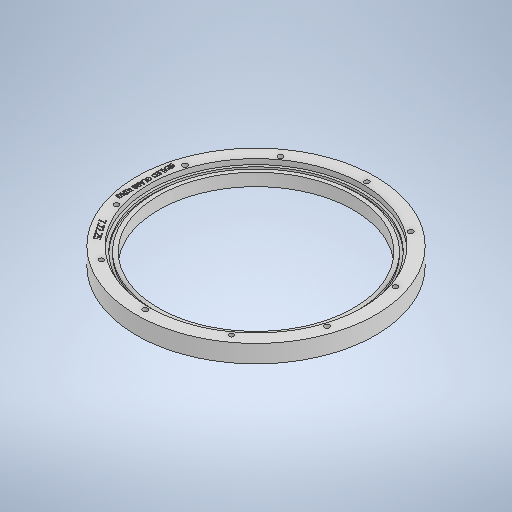
# Autodesk Inventor part: SealedGlassRing
Saved by Autodesk Inventor 2025 (Build 290162000, 162)
## iProperties
Created: 2025-06-19
Part Number: SealedGlassRing
Material: Generic
Document SubType Name: Modeling
Designer: mumin
Density: 1 g/cm^3
Appearance: Default
Author: mumin
Autodesk Inventor part; units mm, degrees
ref_plane "YZ Plane" through (0, 0, 0) normal (1, 0, 0) x (0, 1, 0)
ref_plane "XZ Plane" through (0, 0, 0) normal (0, 1, 0) x (-1, 0, 0)
ref_plane "XY Plane" through (0, 0, 0) normal (0, 0, 1) x (1, 0, 0)
sketch "Sketch1" plane through (0, 0, 0) normal (0, 1, 0) x (-1, 0, 0)
  circle A0 centre (0, 0) radius 110
  circle A1 centre (0, 0) radius 135
  dimension "d0" = 220
  dimension "d1" = 270
  constraints: 2 centre point, 2 coincident
  measures "d0" diameter of A0
  measures "d1" diameter of A1
extrude "Ring" add sketch "Sketch1" along normal blind 20
sketch "Sketch2" plane through (0, 20, 0) normal (0, 1, 0) x (1, 0, 0)
  circle A0 centre (0, 0) radius 120.5
  dimension "d4" = 241
  constraints: 1 centre point, 1 coincident
  measures "d4" diameter of A0
extrude "Glass Seat" cut sketch "Sketch2" against normal blind 5.9
sketch "Sketch3" plane through (0, 20, 0) normal (0, 1, 0) x (1, 0, 0)
  line L0 (0, 189) -> (0, -189) projected
  point P0 (0, 0)
  point P1 (0, 125)
  dimension "d14" = 125
  constraints: 1 point on line
  measures "d14" distance of point (0, 0) point (0, 125)
hole "Holes" at (0, 20, -125) direction (0, -1, 0) diameter 5.5 end through all
pattern_circular "Circular Pattern1" count 10 over 360 about axis through (0, -10, 0) along (0, 1, 0) of "Holes"
sketch "Sketch4" plane through (0, 20, 0) normal (0, 1, 0) x (1, 0, 0)
  line L0 (-123.4008, 33.078) -> (-123.4008, -40.8071) construction
  line L1 (-123.4008, -40.8071) -> (-126.5772, -40.8071) construction
  line L2 (-126.5772, -40.8071) -> (-126.5772, 33.078) construction
  line L3 (-126.5772, 33.078) -> (-123.4008, 33.078) construction
  spline S0 degree 2 poles (-128.5791, 31.1777) (-128.5791, 31.7207) (-128.3522, 32.4824) (-128.1901, 32.8187) knots 0 0 0 1 2 2 2
  line L4 (-128.1901, 32.8187) -> (-127.3554, 32.8187)
  line L5 (-127.3554, 32.8187) -> (-127.3554, 32.7701)
  spline S1 degree 2 poles (-127.3554, 32.7701) (-127.6634, 32.4419) (-128.0037, 31.6113) (-128.0037, 31.2263) knots 0 0 0 1 2 2 2
  spline S2 degree 2 poles (-128.0037, 31.2263) (-128.0037, 30.6753) (-127.5459, 30.1121) (-127.169, 30.1121) knots 0 0 0 1 2 2 2
  spline S3 degree 2 poles (-127.169, 30.1121) (-126.8692, 30.1121) (-126.4964, 30.4079) (-126.4032, 30.7279) knots 0 0 0 1 2 2 2
  spline S4 degree 2 poles (-126.4032, 30.7279) (-126.3384, 30.9589) (-126.2493, 31.3438) (-126.1763, 31.6315) knots 0 0 0 1 2 2 2
  spline S5 degree 2 poles (-126.1763, 31.6315) (-126.1074, 31.8908) (-125.9008, 32.3001) (-125.7347, 32.4581) knots 0 0 0 1 2 2 2
  spline S6 degree 2 poles (-125.7347, 32.4581) (-125.5685, 32.6121) (-125.1228, 32.7822) (-124.8311, 32.7822) knots 0 0 0 1 2 2 2
  spline S7 degree 2 poles (-124.8311, 32.7822) (-124.2233, 32.7822) (-123.4008, 31.8341) (-123.4008, 31.1007) knots 0 0 0 1 2 2 2
  spline S8 degree 2 poles (-123.4008, 31.1007) (-123.4008, 30.6793) (-123.5669, 29.9338) (-123.7249, 29.6137) knots 0 0 0 1 2 2 2
  line L6 (-123.7249, 29.6137) -> (-124.5191, 29.6137)
  line L7 (-124.5191, 29.6137) -> (-124.5191, 29.6623)
  spline S9 degree 2 poles (-124.5191, 29.6623) (-124.3003, 29.9014) (-123.9762, 30.6469) (-123.9762, 31.0561) knots 0 0 0 1 2 2 2
  spline S10 degree 2 poles (-123.9762, 31.0561) (-123.9762, 31.5181) (-124.4097, 32.0894) (-124.7622, 32.0894) knots 0 0 0 1 2 2 2
  spline S11 degree 2 poles (-124.7622, 32.0894) (-125.0783, 32.0894) (-125.4551, 31.7531) (-125.5402, 31.437) knots 0 0 0 1 2 2 2
  spline S12 degree 2 poles (-125.5402, 31.437) (-125.5969, 31.2263) (-125.7428, 30.6145) (-125.8036, 30.4119) knots 0 0 0 1 2 2 2
  spline S13 degree 2 poles (-125.8036, 30.4119) (-125.9616, 29.8973) (-126.5977, 29.4192) (-127.0637, 29.4192) knots 0 0 0 1 2 2 2
  spline S14 degree 2 poles (-127.0637, 29.4192) (-127.3595, 29.4192) (-127.9267, 29.6583) (-128.1253, 29.873) knots 0 0 0 1 2 2 2
  spline S15 degree 2 poles (-128.1253, 29.873) (-128.3441, 30.1121) (-128.5791, 30.7198) (-128.5791, 31.1777) knots 0 0 0 1 2 2 2
  line L8 (-128.4899, 28.7425) -> (-123.4899, 28.7425)
  line L9 (-123.4899, 28.7425) -> (-123.4899, 25.6145)
  line L10 (-123.4899, 25.6145) -> (-124.0815, 25.6145)
  line L11 (-124.0815, 25.6145) -> (-124.0815, 28.078)
  line L12 (-124.0815, 28.078) -> (-125.451, 28.078)
  line L13 (-125.451, 28.078) -> (-125.451, 25.7806)
  line L14 (-125.451, 25.7806) -> (-126.0426, 25.7806)
  line L15 (-126.0426, 25.7806) -> (-126.0426, 28.078)
  line L16 (-126.0426, 28.078) -> (-127.8984, 28.078)
  line L17 (-127.8984, 28.078) -> (-127.8984, 25.6145)
  line L18 (-127.8984, 25.6145) -> (-128.4899, 25.6145)
  line L19 (-128.4899, 25.6145) -> (-128.4899, 28.7425)
  line L20 (-128.4899, 25.4241) -> (-123.4899, 23.7385)
  line L21 (-123.4899, 23.7385) -> (-123.4899, 22.92)
  line L22 (-123.4899, 22.92) -> (-128.4899, 21.2344)
  line L23 (-128.4899, 21.2344) -> (-128.4899, 21.9354)
  line L24 (-128.4899, 21.9354) -> (-127.092, 22.3892)
  line L25 (-127.092, 22.3892) -> (-127.092, 24.2976)
  line L26 (-127.092, 24.2976) -> (-128.4899, 24.7514)
  line L27 (-128.4899, 24.7514) -> (-128.4899, 25.4241)
  line L28 (-126.5248, 22.5715) -> (-124.1707, 23.3455)
  line L29 (-124.1707, 23.3455) -> (-126.5248, 24.1153)
  line L30 (-126.5248, 24.1153) -> (-126.5248, 22.5715)
  line L31 (-128.4899, 17.8633) -> (-128.4899, 20.7604)
  line L32 (-128.4899, 20.7604) -> (-123.4899, 20.7604)
  line L33 (-123.4899, 20.7604) -> (-123.4899, 20.0959)
  line L34 (-123.4899, 20.0959) -> (-127.8984, 20.0959)
  line L35 (-127.8984, 20.0959) -> (-127.8984, 17.8633)
  line L36 (-127.8984, 17.8633) -> (-128.4899, 17.8633)
  line L37 (-128.4899, 17.3406) -> (-123.4899, 17.3406)
  line L38 (-123.4899, 17.3406) -> (-123.4899, 14.2126)
  line L39 (-123.4899, 14.2126) -> (-124.0815, 14.2126)
  line L40 (-124.0815, 14.2126) -> (-124.0815, 16.6761)
  line L41 (-124.0815, 16.6761) -> (-125.451, 16.6761)
  line L42 (-125.451, 16.6761) -> (-125.451, 14.3787)
  line L43 (-125.451, 14.3787) -> (-126.0426, 14.3787)
  line L44 (-126.0426, 14.3787) -> (-126.0426, 16.6761)
  line L45 (-126.0426, 16.6761) -> (-127.8984, 16.6761)
  line L46 (-127.8984, 16.6761) -> (-127.8984, 14.2126)
  line L47 (-127.8984, 14.2126) -> (-128.4899, 14.2126)
  line L48 (-128.4899, 14.2126) -> (-128.4899, 17.3406)
  spline S16 degree 2 poles (-125.994, 9.5408) (-126.6788, 9.5408) (-127.7809, 10.0959) (-128.0888, 10.5618) knots 0 0 0 1 2 2 2
  spline S17 degree 2 poles (-128.0888, 10.5618) (-128.3279, 10.9427) (-128.4899, 11.7247) (-128.4899, 12.3325) knots 0 0 0 1 2 2 2
  line L49 (-128.4899, 12.3325) -> (-128.4899, 13.4832)
  line L50 (-128.4899, 13.4832) -> (-123.4899, 13.4832)
  line L51 (-123.4899, 13.4832) -> (-123.4899, 12.3446)
  spline S18 degree 2 poles (-123.4899, 12.3446) (-123.4899, 11.6396) (-123.7006, 10.8373) (-123.887, 10.5537) knots 0 0 0 1 2 2 2
  spline S19 degree 2 poles (-123.887, 10.5537) (-124.2071, 10.0715) (-125.2647, 9.5408) (-125.994, 9.5408) knots 0 0 0 1 2 2 2
  spline S20 degree 2 poles (-125.9859, 10.2336) (-125.4105, 10.2336) (-124.5961, 10.6145) (-124.3651, 10.9913) knots 0 0 0 1 2 2 2
  spline S21 degree 2 poles (-124.3651, 10.9913) (-124.2071, 11.2587) (-124.0653, 11.8625) (-124.0653, 12.3122) knots 0 0 0 1 2 2 2
  line L52 (-124.0653, 12.3122) -> (-124.0653, 12.8187)
  line L53 (-124.0653, 12.8187) -> (-127.9146, 12.8187)
  line L54 (-127.9146, 12.8187) -> (-127.9146, 12.3122)
  spline S22 degree 2 poles (-127.9146, 12.3122) (-127.9146, 11.8706) (-127.7728, 11.202) (-127.5823, 10.9305) knots 0 0 0 1 2 2 2
  spline S23 degree 2 poles (-127.5823, 10.9305) (-127.3473, 10.5821) (-126.5694, 10.2336) (-125.9859, 10.2336) knots 0 0 0 1 2 2 2
  spline S24 degree 2 poles (-128.5872, 4.5772) (-128.5872, 5.108) (-128.263, 5.9873) (-127.9348, 6.3033) knots 0 0 0 1 2 2 2
  spline S25 degree 2 poles (-127.9348, 6.3033) (-127.6026, 6.6194) (-126.622, 6.9557) (-125.9859, 6.9557) knots 0 0 0 1 2 2 2
  spline S26 degree 2 poles (-125.9859, 6.9557) (-125.3822, 6.9557) (-124.4259, 6.6153) (-124.0856, 6.2993) knots 0 0 0 1 2 2 2
  spline S27 degree 2 poles (-124.0856, 6.2993) (-123.7574, 5.9954) (-123.4008, 5.104) (-123.4008, 4.5732) knots 0 0 0 1 2 2 2
  spline S28 degree 2 poles (-123.4008, 4.5732) (-123.4008, 4.3179) (-123.4737, 3.856) (-123.5386, 3.6453) knots 0 0 0 1 2 2 2
  spline S29 degree 2 poles (-123.5386, 3.6453) (-123.5872, 3.4751) (-123.7655, 3.0618) (-123.8303, 2.9362) knots 0 0 0 1 2 2 2
  line L55 (-123.8303, 2.9362) -> (-124.6326, 2.9362)
  line L56 (-124.6326, 2.9362) -> (-124.6326, 2.9929)
  spline S30 degree 2 poles (-124.6326, 2.9929) (-124.5232, 3.1185) (-124.3246, 3.3819) (-124.2112, 3.625) knots 0 0 0 1 2 2 2
  spline S31 degree 2 poles (-124.2112, 3.625) (-124.1099, 3.8276) (-123.9762, 4.3503) (-123.9762, 4.6502) knots 0 0 0 1 2 2 2
  spline S32 degree 2 poles (-123.9762, 4.6502) (-123.9762, 5.3714) (-125.0621, 6.2628) (-125.9656, 6.2628) knots 0 0 0 1 2 2 2
  spline S33 degree 2 poles (-125.9656, 6.2628) (-126.4681, 6.2628) (-127.2217, 6.0278) (-127.481, 5.8049) knots 0 0 0 1 2 2 2
  spline S34 degree 2 poles (-127.481, 5.8049) (-127.7403, 5.5902) (-128.0118, 4.9824) (-128.0118, 4.6015) knots 0 0 0 1 2 2 2
  spline S35 degree 2 poles (-128.0118, 4.6015) (-128.0118, 4.322) (-127.9308, 3.7628) (-127.8497, 3.5724) knots 0 0 0 1 2 2 2
  line L57 (-127.8497, 3.5724) -> (-126.5572, 3.5724)
  line L58 (-126.5572, 3.5724) -> (-126.5572, 4.7312)
  line L59 (-126.5572, 4.7312) -> (-125.9737, 4.7312)
  line L60 (-125.9737, 4.7312) -> (-125.9737, 2.916)
  line L61 (-125.9737, 2.916) -> (-128.1577, 2.916)
  spline S36 degree 2 poles (-128.1577, 2.916) (-128.2144, 3.0416) (-128.3886, 3.4711) (-128.4413, 3.6534) knots 0 0 0 1 2 2 2
  spline S37 degree 2 poles (-128.4413, 3.6534) (-128.5142, 3.9006) (-128.5872, 4.2976) (-128.5872, 4.5772) knots 0 0 0 1 2 2 2
  line L62 (-128.4899, -0.8158) -> (-128.4899, 2.0813)
  line L63 (-128.4899, 2.0813) -> (-123.4899, 2.0813)
  line L64 (-123.4899, 2.0813) -> (-123.4899, 1.4168)
  line L65 (-123.4899, 1.4168) -> (-127.8984, 1.4168)
  line L66 (-127.8984, 1.4168) -> (-127.8984, -0.8158)
  line L67 (-127.8984, -0.8158) -> (-128.4899, -0.8158)
  line L68 (-128.4899, -0.7996) -> (-123.4899, -2.4852)
  line L69 (-123.4899, -2.4852) -> (-123.4899, -3.3037)
  line L70 (-123.4899, -3.3037) -> (-128.4899, -4.9892)
  line L71 (-128.4899, -4.9892) -> (-128.4899, -4.2883)
  line L72 (-128.4899, -4.2883) -> (-127.092, -3.8345)
  line L73 (-127.092, -3.8345) -> (-127.092, -1.926)
  line L74 (-127.092, -1.926) -> (-128.4899, -1.4722)
  line L75 (-128.4899, -1.4722) -> (-128.4899, -0.7996)
  line L76 (-126.5248, -3.6521) -> (-124.1707, -2.8782)
  line L77 (-124.1707, -2.8782) -> (-126.5248, -2.1084)
  line L78 (-126.5248, -2.1084) -> (-126.5248, -3.6521)
  spline S38 degree 2 poles (-128.5791, -6.8571) (-128.5791, -6.3142) (-128.3522, -5.5524) (-128.1901, -5.2161) knots 0 0 0 1 2 2 2
  line L79 (-128.1901, -5.2161) -> (-127.3554, -5.2161)
  line L80 (-127.3554, -5.2161) -> (-127.3554, -5.2648)
  spline S39 degree 2 poles (-127.3554, -5.2648) (-127.6634, -5.593) (-128.0037, -6.4236) (-128.0037, -6.8085) knots 0 0 0 1 2 2 2
  spline S40 degree 2 poles (-128.0037, -6.8085) (-128.0037, -7.3596) (-127.5459, -7.9228) (-127.169, -7.9228) knots 0 0 0 1 2 2 2
  spline S41 degree 2 poles (-127.169, -7.9228) (-126.8692, -7.9228) (-126.4964, -7.627) (-126.4032, -7.3069) knots 0 0 0 1 2 2 2
  spline S42 degree 2 poles (-126.4032, -7.3069) (-126.3384, -7.0759) (-126.2493, -6.691) (-126.1763, -6.4033) knots 0 0 0 1 2 2 2
  spline S43 degree 2 poles (-126.1763, -6.4033) (-126.1074, -6.144) (-125.9008, -5.7348) (-125.7347, -5.5768) knots 0 0 0 1 2 2 2
  spline S44 degree 2 poles (-125.7347, -5.5768) (-125.5685, -5.4228) (-125.1228, -5.2526) (-124.8311, -5.2526) knots 0 0 0 1 2 2 2
  spline S45 degree 2 poles (-124.8311, -5.2526) (-124.2233, -5.2526) (-123.4008, -6.2007) (-123.4008, -6.9341) knots 0 0 0 1 2 2 2
  spline S46 degree 2 poles (-123.4008, -6.9341) (-123.4008, -7.3555) (-123.5669, -8.1011) (-123.7249, -8.4212) knots 0 0 0 1 2 2 2
  line L81 (-123.7249, -8.4212) -> (-124.5191, -8.4212)
  line L82 (-124.5191, -8.4212) -> (-124.5191, -8.3725)
  spline S47 degree 2 poles (-124.5191, -8.3725) (-124.3003, -8.1335) (-123.9762, -7.3879) (-123.9762, -6.9787) knots 0 0 0 1 2 2 2
  spline S48 degree 2 poles (-123.9762, -6.9787) (-123.9762, -6.5168) (-124.4097, -5.9455) (-124.7622, -5.9455) knots 0 0 0 1 2 2 2
  spline S49 degree 2 poles (-124.7622, -5.9455) (-125.0783, -5.9455) (-125.4551, -6.2818) (-125.5402, -6.5978) knots 0 0 0 1 2 2 2
  spline S50 degree 2 poles (-125.5402, -6.5978) (-125.5969, -6.8085) (-125.7428, -7.4203) (-125.8036, -7.6229) knots 0 0 0 1 2 2 2
  spline S51 degree 2 poles (-125.8036, -7.6229) (-125.9616, -8.1375) (-126.5977, -8.6156) (-127.0637, -8.6156) knots 0 0 0 1 2 2 2
  spline S52 degree 2 poles (-127.0637, -8.6156) (-127.3595, -8.6156) (-127.9267, -8.3766) (-128.1253, -8.1618) knots 0 0 0 1 2 2 2
  spline S53 degree 2 poles (-128.1253, -8.1618) (-128.3441, -7.9228) (-128.5791, -7.315) (-128.5791, -6.8571) knots 0 0 0 1 2 2 2
  spline S54 degree 2 poles (-128.5791, -10.6862) (-128.5791, -10.1432) (-128.3522, -9.3815) (-128.1901, -9.0451) knots 0 0 0 1 2 2 2
  line L83 (-128.1901, -9.0451) -> (-127.3554, -9.0451)
  line L84 (-127.3554, -9.0451) -> (-127.3554, -9.0938)
  spline S55 degree 2 poles (-127.3554, -9.0938) (-127.6634, -9.422) (-128.0037, -10.2526) (-128.0037, -10.6375) knots 0 0 0 1 2 2 2
  spline S56 degree 2 poles (-128.0037, -10.6375) (-128.0037, -11.1886) (-127.5459, -11.7518) (-127.169, -11.7518) knots 0 0 0 1 2 2 2
  spline S57 degree 2 poles (-127.169, -11.7518) (-126.8692, -11.7518) (-126.4964, -11.456) (-126.4032, -11.1359) knots 0 0 0 1 2 2 2
  spline S58 degree 2 poles (-126.4032, -11.1359) (-126.3384, -10.905) (-126.2493, -10.52) (-126.1763, -10.2323) knots 0 0 0 1 2 2 2
  spline S59 degree 2 poles (-126.1763, -10.2323) (-126.1074, -9.973) (-125.9008, -9.5638) (-125.7347, -9.4058) knots 0 0 0 1 2 2 2
  spline S60 degree 2 poles (-125.7347, -9.4058) (-125.5685, -9.2518) (-125.1228, -9.0816) (-124.8311, -9.0816) knots 0 0 0 1 2 2 2
  spline S61 degree 2 poles (-124.8311, -9.0816) (-124.2233, -9.0816) (-123.4008, -10.0298) (-123.4008, -10.7631) knots 0 0 0 1 2 2 2
  spline S62 degree 2 poles (-123.4008, -10.7631) (-123.4008, -11.1845) (-123.5669, -11.9301) (-123.7249, -12.2502) knots 0 0 0 1 2 2 2
  line L85 (-123.7249, -12.2502) -> (-124.5191, -12.2502)
  line L86 (-124.5191, -12.2502) -> (-124.5191, -12.2015)
  spline S63 degree 2 poles (-124.5191, -12.2015) (-124.3003, -11.9625) (-123.9762, -11.2169) (-123.9762, -10.8077) knots 0 0 0 1 2 2 2
  spline S64 degree 2 poles (-123.9762, -10.8077) (-123.9762, -10.3458) (-124.4097, -9.7745) (-124.7622, -9.7745) knots 0 0 0 1 2 2 2
  spline S65 degree 2 poles (-124.7622, -9.7745) (-125.0783, -9.7745) (-125.4551, -10.1108) (-125.5402, -10.4268) knots 0 0 0 1 2 2 2
  spline S66 degree 2 poles (-125.5402, -10.4268) (-125.5969, -10.6375) (-125.7428, -11.2494) (-125.8036, -11.452) knots 0 0 0 1 2 2 2
  spline S67 degree 2 poles (-125.8036, -11.452) (-125.9616, -11.9665) (-126.5977, -12.4447) (-127.0637, -12.4447) knots 0 0 0 1 2 2 2
  spline S68 degree 2 poles (-127.0637, -12.4447) (-127.3595, -12.4447) (-127.9267, -12.2056) (-128.1253, -11.9909) knots 0 0 0 1 2 2 2
  spline S69 degree 2 poles (-128.1253, -11.9909) (-128.3441, -11.7518) (-128.5791, -11.144) (-128.5791, -10.6862) knots 0 0 0 1 2 2 2
  line L87 (-128.4899, -19.1383) -> (-128.4899, -18.2753)
  line L88 (-128.4899, -18.2753) -> (-126.5005, -16.6951)
  line L89 (-126.5005, -16.6951) -> (-126.5005, -15.9333)
  line L90 (-126.5005, -15.9333) -> (-128.4899, -15.9333)
  line L91 (-128.4899, -15.9333) -> (-128.4899, -15.2688)
  line L92 (-128.4899, -15.2688) -> (-123.4899, -15.2688)
  line L93 (-123.4899, -15.2688) -> (-123.4899, -16.5573)
  spline S70 degree 2 poles (-123.4899, -16.5573) (-123.4899, -16.9868) (-123.5831, -17.5662) (-123.7533, -17.8296) knots 0 0 0 1 2 2 2
  spline S71 degree 2 poles (-123.7533, -17.8296) (-123.9235, -18.093) (-124.4543, -18.3968) (-124.8473, -18.3968) knots 0 0 0 1 2 2 2
  spline S72 degree 2 poles (-124.8473, -18.3968) (-125.3943, -18.3968) (-126.1358, -17.8377) (-126.3141, -17.3596) knots 0 0 0 1 2 2 2
  line L94 (-126.3141, -17.3596) -> (-128.4899, -19.1383)
  spline S73 degree 2 poles (-124.9, -17.704) (-124.6812, -17.704) (-124.3449, -17.55) (-124.2355, -17.3879) knots 0 0 0 1 2 2 2
  spline S74 degree 2 poles (-124.2355, -17.3879) (-124.1423, -17.2461) (-124.0653, -16.8693) (-124.0653, -16.5938) knots 0 0 0 1 2 2 2
  line L95 (-124.0653, -16.5938) -> (-124.0653, -15.9333)
  line L96 (-124.0653, -15.9333) -> (-125.9454, -15.9333)
  line L97 (-125.9454, -15.9333) -> (-125.9454, -16.5168)
  spline S75 degree 2 poles (-125.9454, -16.5168) (-125.9454, -16.8045) (-125.8441, -17.2623) (-125.686, -17.4203) knots 0 0 0 1 2 2 2
  spline S76 degree 2 poles (-125.686, -17.4203) (-125.5483, -17.5662) (-125.1593, -17.704) (-124.9, -17.704) knots 0 0 0 1 2 2 2
  line L98 (-128.4899, -21.2777) -> (-128.4899, -19.3409)
  line L99 (-128.4899, -19.3409) -> (-127.9794, -19.3409)
  line L100 (-127.9794, -19.3409) -> (-127.9794, -19.9771)
  line L101 (-127.9794, -19.9771) -> (-124.0005, -19.9771)
  line L102 (-124.0005, -19.9771) -> (-124.0005, -19.3409)
  line L103 (-124.0005, -19.3409) -> (-123.4899, -19.3409)
  line L104 (-123.4899, -19.3409) -> (-123.4899, -21.2777)
  line L105 (-123.4899, -21.2777) -> (-124.0005, -21.2777)
  line L106 (-124.0005, -21.2777) -> (-124.0005, -20.6416)
  line L107 (-124.0005, -20.6416) -> (-127.9794, -20.6416)
  line L108 (-127.9794, -20.6416) -> (-127.9794, -21.2777)
  line L109 (-127.9794, -21.2777) -> (-128.4899, -21.2777)
  line L110 (-128.4899, -25.678) -> (-128.4899, -24.9325)
  line L111 (-128.4899, -24.9325) -> (-124.1788, -22.7202)
  line L112 (-124.1788, -22.7202) -> (-128.4899, -22.7202)
  line L113 (-128.4899, -22.7202) -> (-128.4899, -22.1003)
  line L114 (-128.4899, -22.1003) -> (-123.4899, -22.1003)
  line L115 (-123.4899, -22.1003) -> (-123.4899, -23.0443)
  line L116 (-123.4899, -23.0443) -> (-127.4486, -25.0581)
  line L117 (-127.4486, -25.0581) -> (-123.4899, -25.0581)
  line L118 (-123.4899, -25.0581) -> (-123.4899, -25.678)
  line L119 (-123.4899, -25.678) -> (-128.4899, -25.678)
  spline S77 degree 2 poles (-128.5872, -28.7858) (-128.5872, -28.255) (-128.263, -27.3758) (-127.9348, -27.0597) knots 0 0 0 1 2 2 2
  spline S78 degree 2 poles (-127.9348, -27.0597) (-127.6026, -26.7437) (-126.622, -26.4074) (-125.9859, -26.4074) knots 0 0 0 1 2 2 2
  spline S79 degree 2 poles (-125.9859, -26.4074) (-125.3822, -26.4074) (-124.4259, -26.7477) (-124.0856, -27.0638) knots 0 0 0 1 2 2 2
  spline S80 degree 2 poles (-124.0856, -27.0638) (-123.7574, -27.3677) (-123.4008, -28.2591) (-123.4008, -28.7899) knots 0 0 0 1 2 2 2
  spline S81 degree 2 poles (-123.4008, -28.7899) (-123.4008, -29.0451) (-123.4737, -29.5071) (-123.5386, -29.7178) knots 0 0 0 1 2 2 2
  spline S82 degree 2 poles (-123.5386, -29.7178) (-123.5872, -29.8879) (-123.7655, -30.3012) (-123.8303, -30.4268) knots 0 0 0 1 2 2 2
  line L120 (-123.8303, -30.4268) -> (-124.6326, -30.4268)
  line L121 (-124.6326, -30.4268) -> (-124.6326, -30.3701)
  spline S83 degree 2 poles (-124.6326, -30.3701) (-124.5232, -30.2445) (-124.3246, -29.9811) (-124.2112, -29.738) knots 0 0 0 1 2 2 2
  spline S84 degree 2 poles (-124.2112, -29.738) (-124.1099, -29.5354) (-123.9762, -29.0127) (-123.9762, -28.7129) knots 0 0 0 1 2 2 2
  spline S85 degree 2 poles (-123.9762, -28.7129) (-123.9762, -27.9917) (-125.0621, -27.1003) (-125.9656, -27.1003) knots 0 0 0 1 2 2 2
  spline S86 degree 2 poles (-125.9656, -27.1003) (-126.4681, -27.1003) (-127.2217, -27.3353) (-127.481, -27.5581) knots 0 0 0 1 2 2 2
  spline S87 degree 2 poles (-127.481, -27.5581) (-127.7403, -27.7729) (-128.0118, -28.3806) (-128.0118, -28.7615) knots 0 0 0 1 2 2 2
  spline S88 degree 2 poles (-128.0118, -28.7615) (-128.0118, -29.0411) (-127.9308, -29.6003) (-127.8497, -29.7907) knots 0 0 0 1 2 2 2
  line L122 (-127.8497, -29.7907) -> (-126.5572, -29.7907)
  line L123 (-126.5572, -29.7907) -> (-126.5572, -28.6319)
  line L124 (-126.5572, -28.6319) -> (-125.9737, -28.6319)
  line L125 (-125.9737, -28.6319) -> (-125.9737, -30.4471)
  line L126 (-125.9737, -30.4471) -> (-128.1577, -30.4471)
  spline S89 degree 2 poles (-128.1577, -30.4471) (-128.2144, -30.3215) (-128.3886, -29.892) (-128.4413, -29.7097) knots 0 0 0 1 2 2 2
  spline S90 degree 2 poles (-128.4413, -29.7097) (-128.5142, -29.4625) (-128.5872, -29.0654) (-128.5872, -28.7858) knots 0 0 0 1 2 2 2
  point P0 (0, 0)
  constraints: 2 other
emboss "Emboss1" sketch "Sketch4" operation cut depth 1 direction (0, -1, 0)
sketch "Sketch5" plane through (0, 14.1, 0) normal (0, 1, 0) x (1, 0, 0)
  circle A0 centre (0, 0) radius 120.5 projected
  circle A1 centre (0, 0) radius 117.5
  circle A2 centre (0, 0) radius 114.5
  dimension "d25" = 3
  dimension "d26" = 3
  constraints: 2 centre point
  measures "d25" radial gap between concentric circles of A0 A1
  measures "d26" radial gap between concentric circles of A1 A2
extrude "Seal Groove" cut sketch "Sketch5" against normal blind 2.5 contours A1
sketch "Sketch6" plane through (0, 20, 0) normal (0, 1, 0) x (1, 0, 0)
  line L0 (-109.3924, -58.9981) -> (-82.8013, -97.4436) construction
  line L1 (-82.8013, -97.4436) -> (-85.9073, -99.5919) construction
  line L2 (-85.9073, -99.5919) -> (-112.4984, -61.1464) construction
  line L3 (-112.4984, -61.1464) -> (-109.3924, -58.9981) construction
  line L4 (-107.8437, -63.0408) -> (-113.5155, -63.8067)
  line L5 (-113.5155, -63.8067) -> (-114.0023, -63.1029)
  line L6 (-114.0023, -63.1029) -> (-108.0876, -62.3463)
  line L7 (-108.0876, -62.3463) -> (-109.8494, -59.799)
  line L8 (-109.8494, -59.799) -> (-109.2696, -59.3979)
  line L9 (-109.2696, -59.3979) -> (-107.1039, -62.5291)
  line L10 (-107.1039, -62.5291) -> (-107.8437, -63.0408)
  line L11 (-110.8879, -67.6057) -> (-111.4356, -66.8139)
  line L12 (-111.4356, -66.8139) -> (-110.4918, -66.1612)
  line L13 (-110.4918, -66.1612) -> (-109.9442, -66.953)
  line L14 (-109.9442, -66.953) -> (-110.8879, -67.6057)
  line L15 (-108.0944, -71.6446) -> (-110.1992, -68.6014)
  line L16 (-110.1992, -68.6014) -> (-109.4994, -68.1174)
  spline S0 degree 2 poles (-109.4994, -68.1174) (-108.9647, -68.2323) (-107.989, -68.4207) (-107.4875, -68.4876) knots 0 0 0 1 2 2 2
  spline S1 degree 2 poles (-107.4875, -68.4876) (-106.4777, -68.6227) (-105.449, -68.5202) (-105.0531, -68.2464) knots 0 0 0 1 2 2 2
  spline S2 degree 2 poles (-105.0531, -68.2464) (-104.8452, -68.1025) (-104.6218, -67.7588) (-104.602, -67.5737) knots 0 0 0 1 2 2 2
  spline S3 degree 2 poles (-104.602, -67.5737) (-104.5823, -67.3886) (-104.6925, -67.0155) (-104.8197, -66.8316) knots 0 0 0 1 2 2 2
  spline S4 degree 2 poles (-104.8197, -66.8316) (-104.9414, -66.6556) (-105.2783, -66.3566) (-105.4597, -66.2396) knots 0 0 0 1 2 2 2
  spline S5 degree 2 poles (-105.4597, -66.2396) (-105.6125, -66.1384) (-105.9522, -65.9891) (-106.0635, -65.9479) knots 0 0 0 1 2 2 2
  line L17 (-106.0635, -65.9479) -> (-106.0884, -65.9119)
  line L18 (-106.0884, -65.9119) -> (-105.3846, -65.4251)
  spline S6 degree 2 poles (-105.3846, -65.4251) (-105.1436, -65.5599) (-104.4415, -66.1561) (-104.2147, -66.4841) knots 0 0 0 1 2 2 2
  spline S7 degree 2 poles (-104.2147, -66.4841) (-103.7362, -67.1759) (-103.9286, -68.4618) (-104.5525, -68.8933) knots 0 0 0 1 2 2 2
  spline S8 degree 2 poles (-104.5525, -68.8933) (-104.8444, -69.0952) (-105.4263, -69.2967) (-105.7172, -69.3205) knots 0 0 0 1 2 2 2
  spline S9 degree 2 poles (-105.7172, -69.3205) (-106.0161, -69.3499) (-106.6806, -69.2952) (-107.0174, -69.2443) knots 0 0 0 1 2 2 2
  spline S10 degree 2 poles (-107.0174, -69.2443) (-107.573, -69.1675) (-108.8291, -68.9071) (-109.1987, -68.8257) knots 0 0 0 1 2 2 2
  line L19 (-109.1987, -68.8257) -> (-107.5226, -71.2491)
  line L20 (-107.5226, -71.2491) -> (-108.0944, -71.6446)
  line L21 (-105.5332, -75.3476) -> (-107.638, -72.3044)
  line L22 (-107.638, -72.3044) -> (-106.9382, -71.8204)
  spline S11 degree 2 poles (-106.9382, -71.8204) (-106.4035, -71.9353) (-105.4278, -72.1237) (-104.9263, -72.1906) knots 0 0 0 1 2 2 2
  spline S12 degree 2 poles (-104.9263, -72.1906) (-103.9165, -72.3257) (-102.8878, -72.2232) (-102.4919, -71.9493) knots 0 0 0 1 2 2 2
  spline S13 degree 2 poles (-102.4919, -71.9493) (-102.284, -71.8055) (-102.0606, -71.4618) (-102.0408, -71.2767) knots 0 0 0 1 2 2 2
  spline S14 degree 2 poles (-102.0408, -71.2767) (-102.021, -71.0916) (-102.1313, -70.7185) (-102.2585, -70.5346) knots 0 0 0 1 2 2 2
  spline S15 degree 2 poles (-102.2585, -70.5346) (-102.3802, -70.3586) (-102.7171, -70.0596) (-102.8985, -69.9426) knots 0 0 0 1 2 2 2
  spline S16 degree 2 poles (-102.8985, -69.9426) (-103.0513, -69.8414) (-103.391, -69.6921) (-103.5023, -69.6508) knots 0 0 0 1 2 2 2
  line L23 (-103.5023, -69.6508) -> (-103.5272, -69.6149)
  line L24 (-103.5272, -69.6149) -> (-102.8234, -69.1281)
  spline S17 degree 2 poles (-102.8234, -69.1281) (-102.5824, -69.2629) (-101.8803, -69.8591) (-101.6535, -70.187) knots 0 0 0 1 2 2 2
  spline S18 degree 2 poles (-101.6535, -70.187) (-101.175, -70.8789) (-101.3674, -72.1648) (-101.9913, -72.5963) knots 0 0 0 1 2 2 2
  spline S19 degree 2 poles (-101.9913, -72.5963) (-102.2832, -72.7982) (-102.8651, -72.9997) (-103.156, -73.0235) knots 0 0 0 1 2 2 2
  spline S20 degree 2 poles (-103.156, -73.0235) (-103.4549, -73.0529) (-104.1194, -72.9982) (-104.4562, -72.9473) knots 0 0 0 1 2 2 2
  spline S21 degree 2 poles (-104.4562, -72.9473) (-105.0118, -72.8705) (-106.2679, -72.6101) (-106.6375, -72.5287) knots 0 0 0 1 2 2 2
  line L25 (-106.6375, -72.5287) -> (-104.9614, -74.9521)
  line L26 (-104.9614, -74.9521) -> (-105.5332, -75.3476)
  line L27 (-104.3439, -77.0671) -> (-104.8915, -76.2753)
  line L28 (-104.8915, -76.2753) -> (-103.9478, -75.6226)
  line L29 (-103.9478, -75.6226) -> (-103.4001, -76.4144)
  line L30 (-103.4001, -76.4144) -> (-104.3439, -77.0671)
  line L31 (-101.5503, -81.106) -> (-103.6552, -78.0628)
  line L32 (-103.6552, -78.0628) -> (-102.9554, -77.5788)
  spline S22 degree 2 poles (-102.9554, -77.5788) (-102.4206, -77.6938) (-101.445, -77.8821) (-100.9435, -77.949) knots 0 0 0 1 2 2 2
  spline S23 degree 2 poles (-100.9435, -77.949) (-99.9336, -78.0842) (-98.9049, -77.9816) (-98.5091, -77.7078) knots 0 0 0 1 2 2 2
  spline S24 degree 2 poles (-98.5091, -77.7078) (-98.3011, -77.564) (-98.0777, -77.2202) (-98.0579, -77.0351) knots 0 0 0 1 2 2 2
  spline S25 degree 2 poles (-98.0579, -77.0351) (-98.0382, -76.85) (-98.1484, -76.477) (-98.2756, -76.293) knots 0 0 0 1 2 2 2
  spline S26 degree 2 poles (-98.2756, -76.293) (-98.3973, -76.1171) (-98.7343, -75.818) (-98.9156, -75.7011) knots 0 0 0 1 2 2 2
  spline S27 degree 2 poles (-98.9156, -75.7011) (-99.0684, -75.5998) (-99.4082, -75.4505) (-99.5195, -75.4093) knots 0 0 0 1 2 2 2
  line L33 (-99.5195, -75.4093) -> (-99.5444, -75.3733)
  line L34 (-99.5444, -75.3733) -> (-98.8405, -74.8865)
  spline S28 degree 2 poles (-98.8405, -74.8865) (-98.5995, -75.0213) (-97.8974, -75.6176) (-97.6706, -75.9455) knots 0 0 0 1 2 2 2
  spline S29 degree 2 poles (-97.6706, -75.9455) (-97.1921, -76.6373) (-97.3846, -77.9232) (-98.0084, -78.3547) knots 0 0 0 1 2 2 2
  spline S30 degree 2 poles (-98.0084, -78.3547) (-98.3003, -78.5566) (-98.8822, -78.7581) (-99.1731, -78.7819) knots 0 0 0 1 2 2 2
  spline S31 degree 2 poles (-99.1731, -78.7819) (-99.4721, -78.8113) (-100.1366, -78.7566) (-100.4733, -78.7057) knots 0 0 0 1 2 2 2
  spline S32 degree 2 poles (-100.4733, -78.7057) (-101.0289, -78.6289) (-102.285, -78.3685) (-102.6546, -78.2872) knots 0 0 0 1 2 2 2
  line L35 (-102.6546, -78.2872) -> (-100.9785, -80.7105)
  line L36 (-100.9785, -80.7105) -> (-101.5503, -81.106)
  spline S33 degree 2 poles (-97.4575, -83.6728) (-97.8134, -83.919) (-98.5789, -84.1114) (-98.9467, -84.0584) knots 0 0 0 1 2 2 2
  spline S34 degree 2 poles (-98.9467, -84.0584) (-99.3144, -84.0053) (-100.0031, -83.5653) (-100.2686, -83.1814) knots 0 0 0 1 2 2 2
  spline S35 degree 2 poles (-100.2686, -83.1814) (-100.512, -82.8295) (-100.8318, -82.0338) (-100.8821, -81.6961) knots 0 0 0 1 2 2 2
  line L37 (-100.8821, -81.6961) -> (-100.1822, -81.2121)
  line L38 (-100.1822, -81.2121) -> (-100.1491, -81.2601)
  spline S36 degree 2 poles (-100.1491, -81.2601) (-100.1525, -81.3748) (-100.1001, -81.7583) (-100.0451, -81.9745) knots 0 0 0 1 2 2 2
  spline S37 degree 2 poles (-100.0451, -81.9745) (-99.9776, -82.2175) (-99.8295, -82.5939) (-99.6885, -82.7979) knots 0 0 0 1 2 2 2
  spline S38 degree 2 poles (-99.6885, -82.7979) (-99.5502, -82.9978) (-99.1462, -83.2741) (-98.8962, -83.3022) knots 0 0 0 1 2 2 2
  spline S39 degree 2 poles (-98.8962, -83.3022) (-98.6625, -83.3239) (-98.1821, -83.1808) (-97.9182, -82.9982) knots 0 0 0 1 2 2 2
  spline S40 degree 2 poles (-97.9182, -82.9982) (-97.6543, -82.8157) (-97.4179, -82.4394) (-97.4, -82.226) knots 0 0 0 1 2 2 2
  spline S41 degree 2 poles (-97.4, -82.226) (-97.3728, -82.0003) (-97.5565, -81.5125) (-97.7308, -81.2605) knots 0 0 0 1 2 2 2
  spline S42 degree 2 poles (-97.7308, -81.2605) (-97.9188, -80.9886) (-98.3762, -80.5068) (-98.5256, -80.3678) knots 0 0 0 1 2 2 2
  line L39 (-98.5256, -80.3678) -> (-95.9823, -78.6087)
  line L40 (-95.9823, -78.6087) -> (-94.1098, -81.3159)
  line L41 (-94.1098, -81.3159) -> (-94.6896, -81.717)
  line L42 (-94.6896, -81.717) -> (-96.1224, -79.6456)
  line L43 (-96.1224, -79.6456) -> (-97.438, -80.5555)
  spline S43 degree 2 poles (-97.438, -80.5555) (-97.339, -80.6644) (-97.1666, -80.8881) (-97.1002, -80.984) knots 0 0 0 1 2 2 2
  spline S44 degree 2 poles (-97.1002, -80.984) (-96.8375, -81.3639) (-96.5991, -81.9735) (-96.6171, -82.3407) knots 0 0 0 1 2 2 2
  spline S45 degree 2 poles (-96.6171, -82.3407) (-96.6323, -82.7119) (-97.0096, -83.363) (-97.4575, -83.6728) knots 0 0 0 1 2 2 2
  point P0 (0, 0)
  constraints: 2 other
emboss "Emboss2" sketch "Sketch6" operation cut depth 1 direction (0, -1, 0)
body "Solid1"
